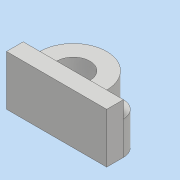
# Autodesk Inventor part: 4
Saved by Autodesk Inventor 2017 (Build 210142000, 142)
## iProperties
Part Number: 4
Material: 一般
Document SubType Name: Modeling
Designer: d8910
Density: 1 g/cm^3
Appearance: 預設
Author: d8910
Autodesk Inventor part; units mm, degrees
ref_plane "YZ Plane" through (0, 0, 0) normal (1, 0, 0) x (0, 1, 0)
ref_plane "XZ Plane" through (0, 0, 0) normal (0, 1, 0) x (-1, 0, 0)
ref_plane "XY Plane" through (0, 0, 0) normal (0, 0, 1) x (1, 0, 0)
sketch "草圖1" plane through (0, 0, 0) normal (0, 0, 1) x (1, 0, 0)
  line L0 (-15, 0) -> (15, 0)
  line L1 (15, 0) -> (15, -5)
  line L2 (15, -5) -> (-15, -5)
  line L3 (-15, -5) -> (-15, 0)
  point P0 (0, 0)
  point P1 (0, -5)
  dimension "d0" = 30
  dimension "d1" = 5
  constraints: 8 end point, 2 parallel, 1 horizontal, 1 horizontal alignment, 1 midpoint, 1 perpendicular, 1 vertical alignment
  measures "d0" distance of L1.end L2.end
  measures "d1" distance of L0.end L1.end
extrude "擠出1" add sketch "草圖1" along normal mid plane 15
sketch "草圖2" plane through (0, 0, -7.5) normal (0, 0, -1) x (-1, 0, 0)
  line L0 (-15, 0) -> (15, 0) construction
  line L1 (15, 0) -> (15, -5) construction
  line L2 (15, -5) -> (-15, -5) construction
  line L3 (-15, -5) -> (-15, 0) construction
  line L4 (-15, 0) -> (-15, 0)
  line L5 (-10, 5) -> (-5, 5)
  line L6 (15, 5) -> (15, 0)
  circle A0 centre (5, 5) radius 5
  arc A1 (15, 5) -> (-5, 5) centre (5, 5) ccw
  line L7 (5, 15) -> (-6.6137, 15) construction
  line L8 (-15, 0) -> (15, 0) projected
  arc A2 (-10, 5) -> (-15, 0) centre (-10, 0) ccw
  line L9 (15, 0) -> (-15, 0)
  point P0 (0, 0)
  dimension "d4" = 5
  dimension "d5" = 10
  dimension "d6" = 15
  dimension "d7" = 10
  dimension "d8" = 5
  constraints: 10 end point, 5 point on circle, 5 tangent, 3 centre point, 2 point on line, 1 coincident, 1 horizontal, 1 parallel
  measures "d4" distance of L6.start L0.end
  measures "d5" radius of A1
  measures "d6" distance between parallel lines of L0 L7
  measures "d7" distance from line of L4 L5.end
  measures "d8" radius of A2
extrude "擠出2" add sketch "草圖2" against normal blind 10
